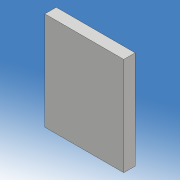
# Autodesk Inventor part: placa_metal
Saved by Autodesk Inventor 2018.3 (Build 223284000, 284)
## iProperties
Created: 2019-03-20
Part Number: placa_metal
Material: Generic
Document SubType Name: Modeling
Designer: vigus
Density: 1 g/cm^3
Appearance: Default
Author: vigus
Autodesk Inventor part; units mm, degrees
ref_plane "YZ Plane" through (0, 0, 0) normal (1, 0, 0) x (0, 1, 0)
ref_plane "XZ Plane" through (0, 0, 0) normal (0, 1, 0) x (-1, 0, 0)
ref_plane "XY Plane" through (0, 0, 0) normal (0, 0, 1) x (1, 0, 0)
sketch "Sketch1" plane through (0, 0, 0) normal (0, 0, 1) x (1, 0, 0)
  line L0 (-22.5, 0) -> (22.5, 0)
  line L1 (22.5, 0) -> (22.5, 6.5)
  line L2 (22.5, 6.5) -> (14.25, 6.5)
  line L3 (14.25, 6.5) -> (14.25, 3.8111)
  line L4 (15.25, 2.8111) -> (18.25, 2.8111)
  line L5 (18.25, 2.8111) -> (18.25, 1.1111)
  line L6 (18.25, 1.1111) -> (12.25, 1.1111)
  line L7 (12.25, 1.1111) -> (12.25, 5)
  line L8 (12.25, 5) -> (-12.25, 5)
  line L9 (-12.25, 5) -> (-12.25, 1.1111)
  line L10 (-12.25, 1.1111) -> (-18.25, 1.1111)
  line L11 (-18.25, 1.1111) -> (-18.25, 2.8111)
  line L12 (-18.25, 2.8111) -> (-15.25, 2.8111)
  line L13 (-14.25, 3.8111) -> (-14.25, 6.5)
  line L14 (-14.25, 6.5) -> (-22.5, 6.5)
  line L15 (-22.5, 6.5) -> (-22.5, 0)
  line L16 (15.25, 2.8111) -> (14.25, 3.8111)
  line L17 (-14.25, 3.8111) -> (-15.25, 2.8111)
  point P0 (0, 0)
  point P1 (14.25, 2.8111)
  point P2 (-14.25, 2.8111)
  dimension "d0" = 45
  dimension "d1" = 6.5
  dimension "d2" = 22.5
  dimension "d3" = 36.5
  dimension "d4" = 4.25
  dimension "d5" = 6
  dimension "d6" = 4
  dimension "d7" = 4
  dimension "d8" = 6
  dimension "d9" = 5
  dimension "d14" = 1.1111
  dimension "d15" = 1.7
  dimension "d16" = 1
  dimension "d17" = 1
  dimension "d18" = 1
  dimension "d19" = 1
  constraints: 36 end point, 11 perpendicular, 10 point on line, 1 horizontal, 1 parallel
  measures "d0" distance of L0.start L0.end
  measures "d1" distance of L0.end L1.end
  measures "d2" distance of point (0, 0) L0.start
  measures "d3" distance between parallel lines of L5 L11
  measures "d4" distance between parallel lines of L15 L11
  measures "d5" distance between parallel lines of L9 L11
  measures "d6" distance of L11.end point (-14.25, 2.811)
  measures "d7" distance of point (14.25, 2.811) L4.end
  measures "d8" distance between parallel lines of L5 L7
  measures "d9" distance between parallel lines of L0 L8
  measures "d14" distance between parallel lines of L0 L6
  measures "d15" distance between parallel lines of L4 L6
  measures "d16" distance of L4.start point (14.25, 2.811)
  measures "d17" distance of L3.end point (14.25, 2.811)
  measures "d18" distance of L13.start point (-14.25, 2.811)
  measures "d19" distance of L12.end point (-14.25, 2.811)
extrude "Extrusion1" add sketch "Sketch1" along normal blind 53
sketch "Sketch2" plane through (0, 0, 53) normal (0, 0, 1) x (1, 0, 0)
  line L0 (-22.5, 0) -> (22.5, 0) projected
  line L1 (-22.5, 6.5) -> (-22.5, 0) projected
  line L2 (22.5, 0) -> (22.5, 6.5) projected
  line L3 (-22.5, 6.5) -> (22.5, 6.5)
  point P0 (0, 0)
  constraints: 2 end point, 1 parallel
extrude "Extrusion2" add sketch "Sketch2" along normal blind 3
equation "\"d17\" = d16"
equation "\"d19\" = d18"
body "Solid1"
